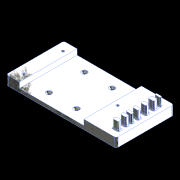
# Autodesk Inventor part: 3d_Welding_Tooling - Adapter
Saved by Autodesk Inventor 2018.3 (Build 223284000, 284)
## iProperties
Created: 2026-01-13
Part Number: 3d_Welding_Tooling - Adapter
Material: Aluminium 6061-T6
Document SubType Name: Modeling
Designer: aca6
Density: 2.7 g/cm^3
Appearance: N/A - Machined Aluminium
Manufacturer-1: {"Name": "Hanstar Technologies Co., Ltd", "PartNumber": "3d_Welding_Tooling - Adapter", "Link": ""}
Manufacturer-2: {"Name": "SHENZHEN JINYIHE PROTOTYPE TECHNOLOGIES CO., LTD", "PartNumber": "3d_Welding_Tooling - Adapter", "Link": ""}
Manufacturer-3: {"Name": "Shenzhen city Xavier Precision Co., Ltd.", "PartNumber": "3d_Welding_Tooling - Adapter", "Link": ""}
Manufacturer-4: {"Name": "", "PartNumber": "", "Link": ""}
Manufacturer-5: {"Name": "", "PartNumber": "", "Link": ""}
Provider-1: {"Name": "", "PartNumber": "", "Link": ""}
Provider-2: {"Name": "", "PartNumber": "", "Link": ""}
Provider-3: {"Name": "", "PartNumber": "", "Link": ""}
Provider-4: {"Name": "", "PartNumber": "", "Link": ""}
Provider-5: {"Name": "", "PartNumber": "", "Link": ""}
Author: aca6
Comments: DIN-ISO-2768-fH
Autodesk Inventor part; units mm, degrees
ref_plane "YZ Plane" through (0, 0, 0) normal (1, 0, 0) x (0, 1, 0)
ref_plane "XZ Plane" through (0, 0, 0) normal (0, 1, 0) x (-1, 0, 0)
ref_plane "XY Plane" through (0, 0, 0) normal (0, 0, 1) x (1, 0, 0)
sketch "Sketch1" plane through (0, 0, 0) normal (0, 0, 1) x (1, 0, 0)
  line L0 (-57.184, 25.25) -> (57.184, 25.25)
  line L1 (57.184, 25.25) -> (57.184, -25.25)
  line L2 (57.184, -25.25) -> (-57.184, -25.25)
  line L3 (-57.184, -25.25) -> (-57.184, 25.25)
  line L4 (0, 0) -> (0, 4.1967) construction
  line L5 (0, 0) -> (4.8916, 0) construction
  dimension "d0" = 114.368
  dimension "d1" = 50.5
  constraints: 12 end point, 3 horizontal, 2 parallel, 2 vertical, 1 perpendicular, 4 other
  measures "d0" distance of L0.start L0.end
  measures "d1" distance of L0.end L1.end
extrude "Extrusion1" add sketch "Sketch1" along normal blind 10
sketch "Sketch2" plane through (0, 0, 10) normal (0, 0, 1) x (1, 0, 0)
  line L0 (57.184, 25.25) -> (-57.184, 25.25) projected
  line L1 (-57.184, 25.25) -> (-57.184, -25.25) projected
  circle A0 centre (-53.184, -21.25) radius 2
  circle A1 centre (-53.184, 21.25) radius 2
  circle A2 centre (27.484, 0) radius 2.5
  circle A3 centre (-53.184, 21.25) radius 1
  circle A4 centre (-53.184, -21.25) radius 1
  circle A5 centre (27.484, 0) radius 1
  point P0 (0, 0)
  dimension "d4" = 42.5
  dimension "d5" = 4
  dimension "d6" = 4
  dimension "d7" = 80.668
  dimension "d8" = 21.25
  dimension "d9" = 4
  dimension "d10" = 4
  dimension "d11" = 5
  dimension "d15" = 2
  dimension "d16" = 2
  dimension "d17" = 2
  constraints: 6 centre point, 6 coincident, 1 vertical alignment
  measures "d4" distance of point (-53.184, 21.25) point (-53.184, -21.25)
  measures "d5" distance from line of L0 point (-53.184, 21.25)
  measures "d6" distance from line of L1 point (-53.184, 21.25)
  measures "d7" horizontal distance of point (-53.184, 21.25) point (27.484, 0)
  measures "d8" vertical distance of point (-53.184, 21.25) point (27.484, 0)
  measures "d9" diameter of A0
  measures "d10" diameter of A1
  measures "d11" diameter of A2
  measures "d15" diameter of A3
  measures "d16" diameter of A4
  measures "d17" diameter of A5
extrude "Extrusion3" cut sketch "Sketch2" against normal blind 5 contours A3 | A4 | A5
ref_plane "Work Plane1" through (-54.684, -25.25, 23) normal (0, 0, -1) x (0, 1, 0)
ref_plane "Work Plane2" through (49.1844, -23.125, 25.1) normal (0, 0, 1) x (1, 0, 0)
sketch "Sketch13" plane through (0, 0, 10) normal (0, 0, 1) x (1, 0, 0)
  line L0 (-41.8192, -14.45) -> (21.1808, -14.45) projected
  line L1 (21.1808, -15.95) -> (21.1808, -14.45) projected
  line L2 (-41.8192, -15.95) -> (21.1808, -15.95) projected
  line L3 (-41.8192, -14.45) -> (-41.8192, -15.95) projected
  line L4 (21.1808, 22.55) -> (-41.8192, 22.55) projected
  line L5 (-41.8192, 24.05) -> (-41.8192, 22.55) projected
  line L6 (-41.8192, 24.05) -> (21.1808, 24.05) projected
  line L7 (21.1808, 22.55) -> (21.1808, 24.05) projected
  line L8 (22.1808, -25.95) -> (-47.8192, -25.95)
  line L9 (-47.8192, -25.95) -> (-47.8192, 25.55)
  line L10 (-47.8192, 25.55) -> (22.1808, 25.55)
  line L11 (22.1808, 25.55) -> (22.1808, -25.95)
  point P0 (0, 0)
  dimension "d52" = 6
  dimension "d53" = 1
  dimension "d54" = 10
  dimension "d55" = 1.5
  constraints: 8 end point, 2 parallel, 1 horizontal, 1 perpendicular
  measures "d52" distance between parallel lines of L5 L9
  measures "d53" distance between parallel lines of L1 L11
  measures "d54" distance between parallel lines of L8 L2
  measures "d55" distance between parallel lines of L6 L10
extrude "Extrusion12" cut sketch "Sketch13" against normal blind 6 contours L0 L1 L2 L3 | L4 L5 L6 L7 | L8 L9 L10 L11
sketch "Sketch17" plane through (-57.184, 25.25, 0) normal (0, 1, 0) x (1, 0, 0)
  line L0 (0, 0) -> (114.368, 0) projected
  line L1 (0, 0) -> (0, -10) projected
  line L2 (9.3648, -10) -> (0, -10) projected
  line L3 (114.368, 0) -> (114.368, -10) projected
  line L4 (79.3648, -4) -> (79.3648, -10) projected
  line L5 (114.368, -10) -> (79.3648, -10) projected
  line L6 (9.3648, -10) -> (9.3648, -4) projected
  line L7 (9.3648, -4) -> (79.3648, -4) projected
  point P0 (57.184, 0)
extrude "Extrusion15" add sketch "Sketch17" along normal blind 6
sketch "Sketch18" plane through (-57.184, -25.25, 0) normal (0, -1, 0) x (1, 0, 0)
  line L0 (114.368, 0) -> (0, 0) projected
  line L1 (114.368, 0) -> (114.368, 10) projected
  line L2 (79.3648, 10) -> (114.368, 10) projected
  line L3 (0, 0) -> (0, 10) projected
  line L4 (79.3648, 10) -> (79.3648, 4) projected
  line L5 (79.3648, 4) -> (9.3648, 4) projected
  line L6 (9.3648, 4) -> (9.3648, 10) projected
  line L7 (0, 10) -> (9.3648, 10) projected
  point P0 (57.184, 0)
extrude "Extrusion16" add sketch "Sketch18" along normal blind 6
sketch "Sketch19" plane through (-57.184, 31.25, 0) normal (-1, 0, 0) x (0, 0, 1)
  line L0 (0, -62.5) -> (0, 0) projected
  line L1 (10, -62.5) -> (0, -62.5) projected
  line L2 (10, -62.5) -> (10, 0) projected
  line L3 (0, 0) -> (10, 0) projected
  point P0 (0, -31.25)
extrude "Extrusion17" add sketch "Sketch19" along normal blind 5
chamfer "Chamfer1" distance 0.5 angle 45 3 edges at (-54.184, -21.25, 10) (-54.184, 21.25, 10) (26.484, 0, 10)
sketch "Sketch20" plane through (0, 0, 10) normal (0, 0, 1) x (1, 0, 0)
  line L0 (46.184, 26.25) -> (52.184, 26.25)
  line L1 (52.184, 26.25) -> (52.184, -26.25)
  line L2 (52.184, -26.25) -> (46.184, -26.25)
  line L3 (46.184, -26.25) -> (46.184, 26.25)
  line L4 (57.184, 31.25) -> (57.184, -31.25) projected
  line L5 (51.6844, 18.625) -> (51.6844, 17.375) construction
  line L6 (51.6844, 17.375) -> (46.6844, 17.375) construction
  line L7 (46.6844, 17.375) -> (46.6844, 18.625) construction
  line L8 (46.6844, 18.625) -> (51.6844, 18.625) construction
  line L9 (46.6844, -23) -> (46.6844, -22) construction
  line L10 (46.6844, -22) -> (51.6844, -22) construction
  line L11 (51.6844, -22) -> (51.6844, -23) construction
  line L12 (51.6844, -23) -> (46.6844, -23) construction
  line L13 (51.6844, 13.9) -> (51.6844, 13.1) construction
  line L14 (51.6844, 13.1) -> (46.6844, 13.1) construction
  line L15 (46.6844, 13.1) -> (46.6844, 13.9) construction
  line L16 (46.6844, 13.9) -> (51.6844, 13.9) construction
  line L17 (51.6844, 10.9) -> (51.6844, 10.1) construction
  line L18 (51.6844, 10.1) -> (46.6844, 10.1) construction
  line L19 (46.6844, 10.1) -> (46.6844, 10.9) construction
  line L20 (46.6844, 10.9) -> (51.6844, 10.9) construction
  line L21 (51.6844, 7.9) -> (51.6844, 7.1) construction
  line L22 (51.6844, 7.1) -> (46.6844, 7.1) construction
  line L23 (46.6844, 7.1) -> (46.6844, 7.9) construction
  line L24 (46.6844, 7.9) -> (51.6844, 7.9) construction
  line L25 (51.6844, 4.9) -> (51.6844, 4.1) construction
  line L26 (51.6844, 4.1) -> (46.6844, 4.1) construction
  line L27 (46.6844, 4.1) -> (46.6844, 4.9) construction
  line L28 (46.6844, 4.9) -> (51.6844, 4.9) construction
  line L29 (51.6844, 1.9) -> (51.6844, 1.1) construction
  line L30 (51.6844, 1.1) -> (46.6844, 1.1) construction
  line L31 (46.6844, 1.1) -> (46.6844, 1.9) construction
  line L32 (46.6844, 1.9) -> (51.6844, 1.9) construction
  line L33 (46.6844, -1.9) -> (46.6844, -1.1) construction
  line L34 (46.6844, -1.1) -> (51.6844, -1.1) construction
  line L35 (51.6844, -1.1) -> (51.6844, -1.9) construction
  line L36 (51.6844, -1.9) -> (46.6844, -1.9) construction
  line L37 (46.6844, -9.4) -> (46.6844, -8.6) construction
  line L38 (46.6844, -8.6) -> (51.6844, -8.6) construction
  line L39 (51.6844, -8.6) -> (51.6844, -9.4) construction
  line L40 (51.6844, -9.4) -> (46.6844, -9.4) construction
  line L41 (51.6844, -11.7) -> (51.6844, -12.5) construction
  line L42 (51.6844, -12.5) -> (46.6844, -12.5) construction
  line L43 (46.6844, -12.5) -> (46.6844, -11.7) construction
  line L44 (46.6844, -11.7) -> (51.6844, -11.7) construction
  line L45 (51.6844, -14.5) -> (51.6844, -15.3) construction
  line L46 (51.6844, -15.3) -> (46.6844, -15.3) construction
  line L47 (46.6844, -15.3) -> (46.6844, -14.5) construction
  line L48 (46.6844, -14.5) -> (51.6844, -14.5) construction
  line L49 (46.6844, -18.4) -> (46.6844, -17.6) construction
  line L50 (46.6844, -17.6) -> (51.6844, -17.6) construction
  line L51 (51.6844, -17.6) -> (51.6844, -18.4) construction
  line L52 (51.6844, -18.4) -> (46.6844, -18.4) construction
  line L53 (46.6844, -19.8) -> (46.6844, -19) construction
  line L54 (46.6844, -19) -> (51.6844, -19) construction
  line L55 (51.6844, -19) -> (51.6844, -19.8) construction
  line L56 (51.6844, -19.8) -> (46.6844, -19.8) construction
  line L57 (46.6844, -17) -> (46.6844, -16.2) construction
  line L58 (46.6844, -16.2) -> (51.6844, -16.2) construction
  line L59 (51.6844, -16.2) -> (51.6844, -17) construction
  line L60 (51.6844, -17) -> (46.6844, -17) construction
  line L61 (51.6844, -13.1) -> (51.6844, -13.9) construction
  line L62 (51.6844, -13.9) -> (46.6844, -13.9) construction
  line L63 (46.6844, -13.9) -> (46.6844, -13.1) construction
  line L64 (46.6844, -13.1) -> (51.6844, -13.1) construction
  line L65 (51.6844, -10) -> (51.6844, -10.8) construction
  line L66 (51.6844, -10.8) -> (46.6844, -10.8) construction
  line L67 (46.6844, -10.8) -> (46.6844, -10) construction
  line L68 (46.6844, -10) -> (51.6844, -10) construction
  line L69 (51.6844, -7.2) -> (51.6844, -8) construction
  line L70 (51.6844, -8) -> (46.6844, -8) construction
  line L71 (46.6844, -8) -> (46.6844, -7.2) construction
  line L72 (46.6844, -7.2) -> (51.6844, -7.2) construction
  line L73 (51.6844, 0.4) -> (51.6844, -0.4) construction
  line L74 (51.6844, -0.4) -> (46.6844, -0.4) construction
  line L75 (46.6844, -0.4) -> (46.6844, 0.4) construction
  line L76 (46.6844, 0.4) -> (51.6844, 0.4) construction
  line L77 (46.6844, 2.6) -> (46.6844, 3.4) construction
  line L78 (46.6844, 3.4) -> (51.6844, 3.4) construction
  line L79 (51.6844, 3.4) -> (51.6844, 2.6) construction
  line L80 (51.6844, 2.6) -> (46.6844, 2.6) construction
  line L81 (51.6844, 6.4) -> (51.6844, 5.6) construction
  line L82 (51.6844, 5.6) -> (46.6844, 5.6) construction
  line L83 (46.6844, 5.6) -> (46.6844, 6.4) construction
  line L84 (46.6844, 6.4) -> (51.6844, 6.4) construction
  line L85 (51.6844, 9.4) -> (51.6844, 8.6) construction
  line L86 (51.6844, 8.6) -> (46.6844, 8.6) construction
  line L87 (46.6844, 8.6) -> (46.6844, 9.4) construction
  line L88 (46.6844, 9.4) -> (51.6844, 9.4) construction
  line L89 (51.6844, 12.4) -> (51.6844, 11.6) construction
  line L90 (51.6844, 11.6) -> (46.6844, 11.6) construction
  line L91 (46.6844, 11.6) -> (46.6844, 12.4) construction
  line L92 (46.6844, 12.4) -> (51.6844, 12.4) construction
  line L93 (46.6844, 14.6) -> (46.6844, 15.4) construction
  line L94 (46.6844, 15.4) -> (51.6844, 15.4) construction
  line L95 (51.6844, 15.4) -> (51.6844, 14.6) construction
  line L96 (51.6844, 14.6) -> (46.6844, 14.6) construction
  line L97 (51.6844, -4) -> (51.6844, -5) construction
  line L98 (51.6844, -5) -> (46.6844, -5) construction
  line L99 (46.6844, -5) -> (46.6844, -4) construction
  line L100 (46.6844, -4) -> (51.6844, -4) construction
  line L101 (46.6844, 21.875) -> (46.6844, 23.125) construction
  line L102 (46.6844, 23.125) -> (51.6844, 23.125) construction
  line L103 (51.6844, 23.125) -> (51.6844, 21.875) construction
  line L104 (51.6844, 21.875) -> (46.6844, 21.875) construction
  circle A0 centre (-53.184, -21.25) radius 1.5 construction
  circle A1 centre (-53.184, 21.25) radius 1.5 construction
  circle A2 centre (27.4844, 0) radius 1.5 construction
  circle A3 centre (-43.1057, -6.1787) radius 0.25 construction
  circle A4 centre (-44.3868, -7.4622) radius 0.25 construction
  circle A5 centre (-44.3868, -4.9219) radius 0.25 construction
  circle A6 centre (-44.3868, -3.6561) radius 0.25 construction
  circle A7 centre (-43.1057, -3.6561) radius 0.25 construction
  circle A8 centre (-44.3868, -6.1787) radius 0.25 construction
  circle A9 centre (-43.1057, -4.9219) radius 0.25 construction
  circle A10 centre (-43.1057, -7.4622) radius 0.25 construction
  circle A11 centre (21.8094, 22) radius 0.35 construction
  circle A12 centre (21.5844, 20) radius 0.825 construction
  circle A13 centre (-47.2156, 20) radius 0.825 construction
  circle A14 centre (18.9844, -22) radius 1.5 construction
  circle A15 centre (-44.6156, -22) radius 1.5 construction
  arc A16 (-56.384, 25.25) -> (-57.184, 24.45) centre (-56.384, 24.45) ccw construction
  line L105 (-57.184, -24.45) -> (-57.184, 24.45) construction
  arc A17 (-57.184, -24.45) -> (-56.384, -25.25) centre (-56.384, -24.45) ccw construction
  line L106 (51.3844, -25.25) -> (-56.384, -25.25) construction
  arc A18 (51.3844, -25.25) -> (52.1844, -24.45) centre (51.3844, -24.45) ccw construction
  line L107 (52.1844, 24.45) -> (52.1844, -24.45) construction
  arc A19 (52.1844, 24.45) -> (51.3844, 25.25) centre (51.3844, 24.45) ccw construction
  line L108 (-56.384, 25.25) -> (51.3844, 25.25) construction
  line L109 (51.6844, 18.625) -> (51.6844, 17.375) construction
  line L110 (51.6844, 17.375) -> (46.6844, 17.375) construction
  line L111 (46.6844, 17.375) -> (46.6844, 18.625) construction
  line L112 (46.6844, 18.625) -> (51.6844, 18.625) construction
  line L113 (46.6844, -23) -> (46.6844, -22) construction
  line L114 (46.6844, -22) -> (51.6844, -22) construction
  line L115 (51.6844, -22) -> (51.6844, -23) construction
  line L116 (51.6844, -23) -> (46.6844, -23) construction
  line L117 (51.6844, 13.9) -> (51.6844, 13.1) construction
  line L118 (51.6844, 13.1) -> (46.6844, 13.1) construction
  line L119 (46.6844, 13.1) -> (46.6844, 13.9) construction
  line L120 (46.6844, 13.9) -> (51.6844, 13.9) construction
  line L121 (51.6844, 10.9) -> (51.6844, 10.1) construction
  line L122 (51.6844, 10.1) -> (46.6844, 10.1) construction
  line L123 (46.6844, 10.1) -> (46.6844, 10.9) construction
  line L124 (46.6844, 10.9) -> (51.6844, 10.9) construction
  line L125 (51.6844, 7.9) -> (51.6844, 7.1) construction
  line L126 (51.6844, 7.1) -> (46.6844, 7.1) construction
  line L127 (46.6844, 7.1) -> (46.6844, 7.9) construction
  line L128 (46.6844, 7.9) -> (51.6844, 7.9) construction
  line L129 (51.6844, 4.9) -> (51.6844, 4.1) construction
  line L130 (51.6844, 4.1) -> (46.6844, 4.1) construction
  line L131 (46.6844, 4.1) -> (46.6844, 4.9) construction
  line L132 (46.6844, 4.9) -> (51.6844, 4.9) construction
  line L133 (51.6844, 1.9) -> (51.6844, 1.1) construction
  line L134 (51.6844, 1.1) -> (46.6844, 1.1) construction
  line L135 (46.6844, 1.1) -> (46.6844, 1.9) construction
  line L136 (46.6844, 1.9) -> (51.6844, 1.9) construction
  line L137 (46.6844, -1.9) -> (46.6844, -1.1) construction
  line L138 (46.6844, -1.1) -> (51.6844, -1.1) construction
  line L139 (51.6844, -1.1) -> (51.6844, -1.9) construction
  line L140 (51.6844, -1.9) -> (46.6844, -1.9) construction
  line L141 (46.6844, -9.4) -> (46.6844, -8.6) construction
  line L142 (46.6844, -8.6) -> (51.6844, -8.6) construction
  line L143 (51.6844, -8.6) -> (51.6844, -9.4) construction
  line L144 (51.6844, -9.4) -> (46.6844, -9.4) construction
  line L145 (51.6844, -11.7) -> (51.6844, -12.5) construction
  line L146 (51.6844, -12.5) -> (46.6844, -12.5) construction
  line L147 (46.6844, -12.5) -> (46.6844, -11.7) construction
  line L148 (46.6844, -11.7) -> (51.6844, -11.7) construction
  line L149 (51.6844, -14.5) -> (51.6844, -15.3) construction
  line L150 (51.6844, -15.3) -> (46.6844, -15.3) construction
  line L151 (46.6844, -15.3) -> (46.6844, -14.5) construction
  line L152 (46.6844, -14.5) -> (51.6844, -14.5) construction
  line L153 (46.6844, -18.4) -> (46.6844, -17.6) construction
  line L154 (46.6844, -17.6) -> (51.6844, -17.6) construction
  line L155 (51.6844, -17.6) -> (51.6844, -18.4) construction
  line L156 (51.6844, -18.4) -> (46.6844, -18.4) construction
  line L157 (46.6844, -19.8) -> (46.6844, -19) construction
  line L158 (46.6844, -19) -> (51.6844, -19) construction
  line L159 (51.6844, -19) -> (51.6844, -19.8) construction
  line L160 (51.6844, -19.8) -> (46.6844, -19.8) construction
  line L161 (46.6844, -17) -> (46.6844, -16.2) construction
  line L162 (46.6844, -16.2) -> (51.6844, -16.2) construction
  line L163 (51.6844, -16.2) -> (51.6844, -17) construction
  line L164 (51.6844, -17) -> (46.6844, -17) construction
  line L165 (51.6844, -13.1) -> (51.6844, -13.9) construction
  line L166 (51.6844, -13.9) -> (46.6844, -13.9) construction
  line L167 (46.6844, -13.9) -> (46.6844, -13.1) construction
  line L168 (46.6844, -13.1) -> (51.6844, -13.1) construction
  line L169 (51.6844, -10) -> (51.6844, -10.8) construction
  line L170 (51.6844, -10.8) -> (46.6844, -10.8) construction
  line L171 (46.6844, -10.8) -> (46.6844, -10) construction
  line L172 (46.6844, -10) -> (51.6844, -10) construction
  line L173 (51.6844, -7.2) -> (51.6844, -8) construction
  line L174 (51.6844, -8) -> (46.6844, -8) construction
  line L175 (46.6844, -8) -> (46.6844, -7.2) construction
  line L176 (46.6844, -7.2) -> (51.6844, -7.2) construction
  line L177 (51.6844, 0.4) -> (51.6844, -0.4) construction
  line L178 (51.6844, -0.4) -> (46.6844, -0.4) construction
  line L179 (46.6844, -0.4) -> (46.6844, 0.4) construction
  line L180 (46.6844, 0.4) -> (51.6844, 0.4) construction
  line L181 (46.6844, 2.6) -> (46.6844, 3.4) construction
  line L182 (46.6844, 3.4) -> (51.6844, 3.4) construction
  line L183 (51.6844, 3.4) -> (51.6844, 2.6) construction
  line L184 (51.6844, 2.6) -> (46.6844, 2.6) construction
  line L185 (51.6844, 6.4) -> (51.6844, 5.6) construction
  line L186 (51.6844, 5.6) -> (46.6844, 5.6) construction
  line L187 (46.6844, 5.6) -> (46.6844, 6.4) construction
  line L188 (46.6844, 6.4) -> (51.6844, 6.4) construction
  line L189 (51.6844, 9.4) -> (51.6844, 8.6) construction
  line L190 (51.6844, 8.6) -> (46.6844, 8.6) construction
  line L191 (46.6844, 8.6) -> (46.6844, 9.4) construction
  line L192 (46.6844, 9.4) -> (51.6844, 9.4) construction
  line L193 (51.6844, 12.4) -> (51.6844, 11.6) construction
  line L194 (51.6844, 11.6) -> (46.6844, 11.6) construction
  line L195 (46.6844, 11.6) -> (46.6844, 12.4) construction
  line L196 (46.6844, 12.4) -> (51.6844, 12.4) construction
  line L197 (46.6844, 14.6) -> (46.6844, 15.4) construction
  line L198 (46.6844, 15.4) -> (51.6844, 15.4) construction
  line L199 (51.6844, 15.4) -> (51.6844, 14.6) construction
  line L200 (51.6844, 14.6) -> (46.6844, 14.6) construction
  line L201 (51.6844, -4) -> (51.6844, -5) construction
  line L202 (51.6844, -5) -> (46.6844, -5) construction
  line L203 (46.6844, -5) -> (46.6844, -4) construction
  line L204 (46.6844, -4) -> (51.6844, -4) construction
  line L205 (46.6844, 21.875) -> (46.6844, 23.125) construction
  line L206 (46.6844, 23.125) -> (51.6844, 23.125) construction
  line L207 (51.6844, 23.125) -> (51.6844, 21.875) construction
  line L208 (51.6844, 21.875) -> (46.6844, 21.875) construction
  circle A20 centre (-53.184, -21.25) radius 1.5 construction
  circle A21 centre (-53.184, 21.25) radius 1.5 construction
  circle A22 centre (27.4844, 0) radius 1.5 construction
  circle A23 centre (-43.1057, -6.1787) radius 0.25 construction
  circle A24 centre (-44.3868, -7.4622) radius 0.25 construction
  circle A25 centre (-44.3868, -4.9219) radius 0.25 construction
  circle A26 centre (-44.3868, -3.6561) radius 0.25 construction
  circle A27 centre (-43.1057, -3.6561) radius 0.25 construction
  circle A28 centre (-44.3868, -6.1787) radius 0.25 construction
  circle A29 centre (-43.1057, -4.9219) radius 0.25 construction
  circle A30 centre (-43.1057, -7.4622) radius 0.25 construction
  circle A31 centre (21.8094, 22) radius 0.35 construction
  circle A32 centre (21.5844, 20) radius 0.825 construction
  circle A33 centre (-47.2156, 20) radius 0.825 construction
  circle A34 centre (18.9844, -22) radius 1.5 construction
  circle A35 centre (-44.6156, -22) radius 1.5 construction
  arc A36 (-56.384, 25.25) -> (-57.184, 24.45) centre (-56.384, 24.45) ccw construction
  line L209 (-57.184, -24.45) -> (-57.184, 24.45) construction
  arc A37 (-57.184, -24.45) -> (-56.384, -25.25) centre (-56.384, -24.45) ccw construction
  line L210 (51.3844, -25.25) -> (-56.384, -25.25) construction
  arc A38 (51.3844, -25.25) -> (52.1844, -24.45) centre (51.3844, -24.45) ccw construction
  line L211 (52.1844, 24.45) -> (52.1844, -24.45) construction
  arc A39 (52.1844, 24.45) -> (51.3844, 25.25) centre (51.3844, 24.45) ccw construction
  line L212 (-56.384, 25.25) -> (51.3844, 25.25) construction
  line L213 (52.1844, -14) -> (52.1844, -13)
  line L214 (46.184, 4) -> (46.184, 5)
  line L215 (46.184, -24) -> (52.1844, -24)
  line L216 (46.184, -20.5) -> (52.1844, -20.5)
  line L217 (46.184, -15.6851) -> (52.1844, -15.6851)
  line L218 (46.184, -12.1851) -> (52.1844, -12.1851)
  line L219 (46.1827, -6.9016) -> (52.1831, -6.9016)
  line L220 (46.1827, -9.7016) -> (52.1831, -9.7016)
  line L221 (52.1844, -2.6369) -> (46.184, -2.6369)
  line L222 (52.1844, 0.6631) -> (46.184, 0.6631)
  line L223 (46.184, 6) -> (52.1844, 6)
  line L224 (46.184, 9.6) -> (52.1844, 9.6)
  line L225 (46.184, 14.5092) -> (52.1844, 14.5092)
  line L226 (46.184, 18.7092) -> (52.1844, 18.7092)
  line L227 (46.184, 21.4636) -> (52.1844, 21.4636)
  line L228 (46.184, 23.4636) -> (52.1844, 23.4636)
  line L229 (52.1844, -15.6851) -> (52.1844, -12.1851)
  line L230 (46.184, -15.6851) -> (46.184, -12.1851)
  line L231 (46.1827, -9.7016) -> (46.1827, -6.9016)
  line L232 (52.1831, -9.7016) -> (52.1831, -6.9016)
  line L233 (52.1844, -2.6369) -> (52.1844, 0.6631)
  line L234 (46.184, -2.6369) -> (46.184, 0.6631)
  line L235 (46.184, 6) -> (46.184, 9.6)
  line L236 (52.1844, 6) -> (52.1844, 9.6)
  line L237 (46.184, 14.5092) -> (46.184, 18.7092)
  line L238 (52.1844, 14.5092) -> (52.1844, 18.7092)
  line L239 (52.1844, 21.4636) -> (52.1844, 23.4636)
  line L240 (46.184, 21.4636) -> (46.184, 23.4636)
  line L241 (52.1844, -24) -> (52.1844, -20.5)
  line L242 (46.184, -24) -> (46.184, -20.5)
  point P0 (0, 0)
  dimension "d88" = 6
  dimension "d89" = 11
  dimension "d91" = 1
  dimension "d92" = 1
  dimension "d113" = 3.5
  dimension "d116" = 3.5
  dimension "d119" = 2.8
  dimension "d120" = 3.3
  dimension "d122" = 4.2
  dimension "d123" = 2
  dimension "d124" = 10.5649
  dimension "d127" = 16.5484
  dimension "d128" = 23.6131
  dimension "d130" = 11.7408
  dimension "d131" = 4.7864
  dimension "d132" = 1
  dimension "d133" = 0.4
  dimension "d134" = 5.75
  constraints: 68 end point, 17 parallel, 11 point on line, 8 perpendicular, 6 collinear, 2 horizontal
  measures "d88" distance between parallel lines of L1 L3
  measures "d89" distance between parallel lines of L4 L3
  measures "d91" distance between parallel lines of L106 L2
  measures "d92" distance between parallel lines of L108 L0
  measures "d113" distance between parallel lines of L215 L216
  measures "d116" distance between parallel lines of L218 L217
  measures "d119" distance between parallel lines of L219 L220
  measures "d120" distance between parallel lines of L221 L222
  measures "d122" distance between parallel lines of L225 L226
  measures "d123" distance between parallel lines of L227 L228
  measures "d124" distance between parallel lines of L2 L217
  measures "d127" distance between parallel lines of L2 L220
  measures "d128" distance between parallel lines of L2 L221
  measures "d130" distance between parallel lines of L0 L225
  measures "d131" distance between parallel lines of L0 L227
  measures "d132" distance between parallel lines of L190 L224
  measures "d133" distance between parallel lines of L188 L223
  measures "d134" distance between parallel lines of L2 L216
extrude "Extrusion18" add sketch "Sketch20" along normal blind 9 contours L228 L1 L227 L3 | L226 L1 L225 L3 | L224 L1 L223 L3 | L1 L221 L3 L222 | L1 L220 L3 L219 | L1 L217 L3 L218 | L216 L1 L215 L3
fillet "Fillet11" radius 1 8 edges at (52.1844, -24, 14.5) (52.1844, -20.5, 14.5) (46.184, -24, 14.5) (46.184, -20.5, 14.5) (52.1844, -22.25, 10) (49.1842, -24, 10) (49.1842, -20.5, 10) (46.184, -22.25, 10)
fillet "Fillet11" radius 1 8 edges at (52.1844, -15.6851, 14.5) (52.1844, -12.1851, 14.5) (52.1844, -13.9351, 10) (46.184, -15.6851, 14.5) (49.1842, -15.6851, 10) (49.1842, -12.1851, 10) (46.184, -12.1851, 14.5) (46.184, -13.9351, 10)
fillet "Fillet11" radius 1 8 edges at (52.1831, -8.3016, 10) (49.1829, -9.7016, 10) (52.1831, -9.7016, 14.5) (52.1831, -6.9016, 14.5) (46.1827, -9.7016, 14.5) (46.1827, -6.9016, 14.5) (49.1829, -6.9016, 10) (46.1827, -8.3016, 10)
fillet "Fillet11" radius 1 8 edges at (52.1844, -0.9869, 10) (52.1844, -2.6369, 14.5) (52.1844, 0.6631, 14.5) (49.1842, 0.6631, 10) (46.184, 0.6631, 14.5) (46.184, -2.6369, 14.5) (49.1842, -2.6369, 10) (46.184, -0.9869, 10)
fillet "Fillet11" radius 1 8 edges at (52.1844, 7.8, 10) (49.1842, 9.6, 10) (52.1844, 9.6, 14.5) (52.1844, 6, 14.5) (46.184, 9.6, 14.5) (46.184, 7.8, 10) (46.184, 6, 14.5) (49.1842, 6, 10)
fillet "Fillet11" radius 1 8 edges at (52.1844, 16.6092, 10) (52.1844, 14.5092, 14.5) (52.1844, 18.7092, 14.5) (49.1842, 18.7092, 10) (46.184, 18.7092, 14.5) (49.1842, 14.5092, 10) (46.184, 14.5092, 14.5) (46.184, 16.6092, 10)
fillet "Fillet12" radius 0.7 8 edges at (49.1842, 23.4636, 10) (49.1842, 21.4636, 10) (52.1844, 22.4636, 10) (52.1844, 21.4636, 14.5) (52.1844, 23.4636, 14.5) (46.184, 22.4636, 10) (46.184, 23.4636, 14.5) (46.184, 21.4636, 14.5)
fillet "Fillet13" radius 2 4 edges at (-62.184, -31.25, 5) (57.184, -31.25, 5) (57.184, 31.25, 5) (-62.184, 31.25, 5)
sketch "Sketch21" plane through (0, 0, 4) normal (0, 0, 1) x (1, 0, 0)
  line L0 (-47.8192, 31.25) -> (22.1808, 31.25) projected
  line L1 (22.1808, -31.25) -> (-47.8192, -31.25) projected
  line L2 (-47.8192, -31.25) -> (-47.8192, 31.25) projected
  line L3 (22.1808, 31.25) -> (22.1808, -31.25) projected
  circle A0 centre (2.1808, 19.25) radius 3
  circle A1 centre (-27.8192, 19.25) radius 3
  circle A2 centre (-27.8192, -19.25) radius 3
  circle A3 centre (2.1808, -19.25) radius 3
  point P0 (0, 0)
  dimension "d144" = 12
  dimension "d145" = 12
  dimension "d146" = 12
  dimension "d147" = 12
  dimension "d148" = 20
  dimension "d149" = 20
  dimension "d150" = 20
  dimension "d151" = 20
  dimension "d152" = 6
  dimension "d153" = 6
  dimension "d154" = 6
  dimension "d155" = 6
  constraints: 4 centre point, 4 coincident
  measures "d144" distance from line of point (-27.819, 19.25) L0
  measures "d145" distance from line of L0 point (2.181, 19.25)
  measures "d146" distance from line of L1 point (2.181, -19.25)
  measures "d147" distance from line of L1 point (-27.819, -19.25)
  measures "d148" distance from line of L2 point (-27.819, -19.25)
  measures "d149" distance from line of L3 point (2.181, -19.25)
  measures "d150" distance from line of L3 point (2.181, 19.25)
  measures "d151" distance from line of L2 point (-27.819, 19.25)
  measures "d152" diameter of A0
  measures "d153" diameter of A1
  measures "d154" diameter of A2
  measures "d155" diameter of A3
extrude "Extrusion19" cut sketch "Sketch21" against normal blind 0.3 contours A0 | A1 | A2 | A3
sketch "Sketch22" plane through (-27.8192, -19.25, 3.7) normal (0, 0, 1) x (1, 0, 0)
  circle A0 centre (30, 38.5) radius 3 projected
  circle A1 centre (30, 0) radius 3 projected
  circle A2 centre (0, 0) radius 3 projected
  circle A3 centre (0, 38.5) radius 3 projected
  point P0 (27.8192, 19.25)
  constraints: 4 coincident
hole "Hole1" at (2.1808, 19.25, 3.7) at (2.1808, -19.25, 3.7) at (-27.8192, -19.25, 3.7) at (-27.8192, 19.25, 3.7) direction (0, 0, -1) diameter 3.2 depth 8 tip angle 118 countersink diameter 6 countersink angle 90
body "Solid1"
